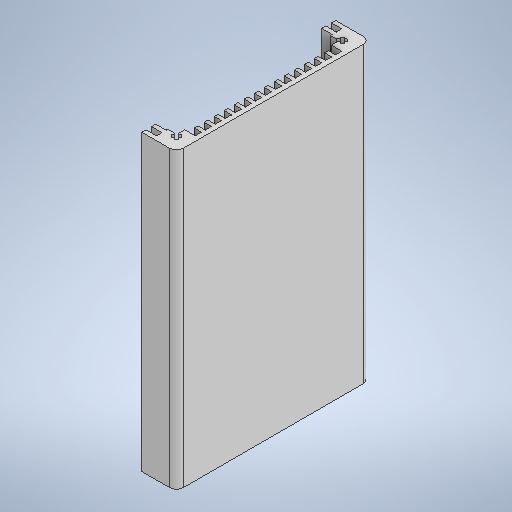
# Autodesk Inventor part: Side Section 2
Saved by Autodesk Inventor 2025 (Build 290162000, 162)
## iProperties
Created: 2024-06-11
Part Number: Side Section 2
Material: Generic
Document SubType Name: Modeling
Designer: Caleb Fangmeier
Density: 1 g/cm^3
Appearance: Default
Author: Caleb Fangmeier
Autodesk Inventor part; units mm, degrees
ref_plane "YZ Plane" through (0, 0, 0) normal (1, 0, 0) x (0, 1, 0)
ref_plane "XZ Plane" through (0, 0, 0) normal (0, 1, 0) x (-1, 0, 0)
ref_plane "XY Plane" through (0, 0, 0) normal (0, 0, 1) x (1, 0, 0)
sketch "Sketch1" plane through (0, 0, 0) normal (0, 1, 0) x (-1, 0, 0)
  line L0 (0, 28) -> (0, -28)
  line L1 (0, 28) -> (10, 28)
  line L2 (0, 28) -> (10, 28) construction
  line L3 (10, 28) -> (10, 26.8)
  line L4 (10, 26.8) -> (7, 26.8)
  line L5 (7, 26.8) -> (7, 25.2)
  line L6 (7, 25.2) -> (10, 25.2)
  line L7 (10, 25.2) -> (10, 24)
  line L8 (10, 24) -> (7, 24)
  line L9 (2.9393, 24.3536) -> (3.6464, 25.0607)
  line L10 (2.9393, 24.3536) -> (3.9393, 24.3536) construction
  line L11 (3.6464, 25.0607) -> (4, 24.7071)
  line L12 (4, 24.7071) -> (4.3536, 25.0607)
  line L13 (4.3536, 25.0607) -> (5.0607, 24.3536)
  line L14 (5.0607, 24.3536) -> (4.7071, 24)
  line L15 (2.9393, 24.3536) -> (3.2929, 24)
  line L16 (3.2929, 24) -> (2.9393, 23.6464)
  line L17 (2.9393, 23.6464) -> (3.6464, 22.9393)
  line L18 (3.6464, 22.9393) -> (4, 23.2929)
  line L19 (4.7071, 24) -> (5.2071, 23.5)
  line L20 (4, 23.2929) -> (4.3536, 22.9393)
  line L21 (7, 24) -> (7, 23.5)
  line L22 (7, 23.5) -> (5.2071, 23.5)
  line L23 (1.4, 0) -> (1.4, 0.9)
  line L24 (1.4, 0.9) -> (3.5, 0.9)
  line L25 (3.5, 0.9) -> (3.5, 2)
  line L26 (3.5, 2) -> (1.4, 2)
  line L27 (1.4, 2) -> (1.4, 2.9)
  line L28 (1.4, 2.9) -> (1.4, 3.8)
  line L29 (1.4, 3.8) -> (3.5, 3.8)
  line L30 (3.5, 3.8) -> (3.5, 4.9)
  line L31 (3.5, 4.9) -> (1.4, 4.9)
  line L32 (1.4, 4.9) -> (1.4, 5.8)
  line L33 (1.4, 5.8) -> (1.4, 6.7)
  line L34 (1.4, 6.7) -> (3.5, 6.7)
  line L35 (3.5, 6.7) -> (3.5, 7.8)
  line L36 (3.5, 7.8) -> (1.4, 7.8)
  line L37 (1.4, 7.8) -> (1.4, 8.7)
  line L38 (1.4, 8.7) -> (1.4, 9.6)
  line L39 (1.4, 9.6) -> (3.5, 9.6)
  line L40 (3.5, 9.6) -> (3.5, 10.7)
  line L41 (3.5, 10.7) -> (1.4, 10.7)
  line L42 (1.4, 10.7) -> (1.4, 11.6)
  line L43 (1.4, 11.6) -> (1.4, 12.5)
  line L44 (1.4, 12.5) -> (3.5, 12.5)
  line L45 (3.5, 12.5) -> (3.5, 13.6)
  line L46 (3.5, 13.6) -> (1.4, 13.6)
  line L47 (1.4, 13.6) -> (1.4, 14.5)
  line L48 (1.4, 14.5) -> (1.4, 15.4)
  line L49 (1.4, 15.4) -> (3.5, 15.4)
  line L50 (3.5, 15.4) -> (3.5, 16.5)
  line L51 (3.5, 16.5) -> (1.4, 16.5)
  line L52 (1.4, 16.5) -> (1.4, 17.4)
  line L53 (1.4, 17.4) -> (1.4, 18.3)
  line L54 (1.4, 18.3) -> (3.5, 18.3)
  line L55 (3.5, 18.3) -> (3.5, 19.4)
  line L56 (3.5, 19.4) -> (1.4, 19.4)
  line L57 (1.4, 19.4) -> (1.4, 20.3)
  line L58 (1.4, 20.3) -> (1.4, 21.2)
  line L59 (1.4, 21.2) -> (4.4, 21.2)
  line L60 (4.4, 21.2) -> (4.4, 22.8929)
  line L61 (4.4, 22.8929) -> (4.3536, 22.9393)
  line L62 (13.8128, 0) -> (-10.738, 0)
  line L63 (0, -28) -> (10, -28)
  line L64 (0, -28) -> (10, -28) construction
  line L65 (10, -28) -> (10, -26.8)
  line L66 (10, -26.8) -> (7, -26.8)
  line L67 (7, -26.8) -> (7, -25.2)
  line L68 (7, -25.2) -> (10, -25.2)
  line L69 (10, -25.2) -> (10, -24)
  line L70 (10, -24) -> (7, -24)
  line L71 (2.9393, -24.3536) -> (3.6464, -25.0607)
  line L72 (2.9393, -24.3536) -> (3.9393, -24.3536) construction
  line L73 (3.6464, -25.0607) -> (4, -24.7071)
  line L74 (4, -24.7071) -> (4.3536, -25.0607)
  line L75 (4.3536, -25.0607) -> (5.0607, -24.3536)
  line L76 (5.0607, -24.3536) -> (4.7071, -24)
  line L77 (2.9393, -24.3536) -> (3.2929, -24)
  line L78 (3.2929, -24) -> (2.9393, -23.6464)
  line L79 (2.9393, -23.6464) -> (3.6464, -22.9393)
  line L80 (3.6464, -22.9393) -> (4, -23.2929)
  line L81 (4.7071, -24) -> (5.2071, -23.5)
  line L82 (4, -23.2929) -> (4.3536, -22.9393)
  line L83 (7, -24) -> (7, -23.5)
  line L84 (7, -23.5) -> (5.2071, -23.5)
  line L85 (1.4, 0) -> (1.4, -0.9)
  line L86 (1.4, -0.9) -> (3.5, -0.9)
  line L87 (3.5, -0.9) -> (3.5, -2)
  line L88 (3.5, -2) -> (1.4, -2)
  line L89 (1.4, -2) -> (1.4, -2.9)
  line L90 (1.4, -2.9) -> (1.4, -3.8)
  line L91 (1.4, -3.8) -> (3.5, -3.8)
  line L92 (3.5, -3.8) -> (3.5, -4.9)
  line L93 (3.5, -4.9) -> (1.4, -4.9)
  line L94 (1.4, -4.9) -> (1.4, -5.8)
  line L95 (1.4, -5.8) -> (1.4, -6.7)
  line L96 (1.4, -6.7) -> (3.5, -6.7)
  line L97 (3.5, -6.7) -> (3.5, -7.8)
  line L98 (3.5, -7.8) -> (1.4, -7.8)
  line L99 (1.4, -7.8) -> (1.4, -8.7)
  line L100 (1.4, -8.7) -> (1.4, -9.6)
  line L101 (1.4, -9.6) -> (3.5, -9.6)
  line L102 (3.5, -9.6) -> (3.5, -10.7)
  line L103 (3.5, -10.7) -> (1.4, -10.7)
  line L104 (1.4, -10.7) -> (1.4, -11.6)
  line L105 (1.4, -11.6) -> (1.4, -12.5)
  line L106 (1.4, -12.5) -> (3.5, -12.5)
  line L107 (3.5, -12.5) -> (3.5, -13.6)
  line L108 (3.5, -13.6) -> (1.4, -13.6)
  line L109 (1.4, -13.6) -> (1.4, -14.5)
  line L110 (1.4, -14.5) -> (1.4, -15.4)
  line L111 (1.4, -15.4) -> (3.5, -15.4)
  line L112 (3.5, -15.4) -> (3.5, -16.5)
  line L113 (3.5, -16.5) -> (1.4, -16.5)
  line L114 (1.4, -16.5) -> (1.4, -17.4)
  line L115 (1.4, -17.4) -> (1.4, -18.3)
  line L116 (1.4, -18.3) -> (3.5, -18.3)
  line L117 (3.5, -18.3) -> (3.5, -19.4)
  line L118 (3.5, -19.4) -> (1.4, -19.4)
  line L119 (1.4, -19.4) -> (1.4, -20.3)
  line L120 (1.4, -20.3) -> (1.4, -21.2)
  line L121 (1.4, -21.2) -> (4.4, -21.2)
  line L122 (4.4, -21.2) -> (4.4, -22.8929)
  line L123 (4.4, -22.8929) -> (4.3536, -22.9393)
  point P0 (0, 0)
  point P1 (4, 24)
  point P2 (0, 0)
  point P3 (4, -24)
  dimension "d0" = 56
  dimension "d1" = 10
  dimension "d3" = 28
  dimension "d4" = 1.2
  dimension "d5" = 3
  dimension "d6" = 1.6
  dimension "d7" = 1.2
  dimension "d9" = 24
  dimension "d10" = 4
  dimension "d11" = 1
  dimension "d12" = 45
  dimension "d13" = 1
  dimension "d14" = 1
  dimension "d15" = 0.5
  dimension "d16" = 0.5
  dimension "d17" = 0.5
  dimension "d18" = 0.5
  dimension "d20" = 0.5
  dimension "d21" = 0.5
  dimension "d25" = 0.9
  dimension "d26" = 1.4
  dimension "d27" = 2.1
  dimension "d28" = 1.1
  dimension "d29" = 0.9
  dimension "d32" = 2.9
  dimension "d37" = 0.9
  dimension "d38" = 3
  constraints: 248 end point, 67 symmetric about line, 15 perpendicular, 10 point on line, 7 vertical, 6 horizontal, 3 vertical alignment, 2 equal length, 2 horizontal alignment, 2 midpoint, 1 parallel, 66 other
  measures "d0" distance of L0.start L0.end
  measures "d1" distance of L0.start L1.end
  measures "d3" distance of L0.start point (0, 0)
  measures "d4" distance of L2.end L3.end
  measures "d5" distance of L3.end L4.end
  measures "d6" distance of L4.end L5.end
  measures "d7" distance of L6.end L7.end
  measures "d9" vertical distance of point (4, 24) point (0, 0)
  measures "d10" horizontal distance of point (0, 0) point (4, 24)
  measures "d11" distance of L9.start L9.end
  measures "d12" angle of L10 L9
  measures "d13" distance of L12.end L13.end
  measures "d14" distance of L16.end L17.end
  measures "d15" distance of L9.start L15.end
  measures "d16" distance of L9.end L11.end
  measures "d17" distance of L13.end L14.end
  measures "d18" distance of L17.end L18.end
  measures "d20" distance of L18.end L20.end
  measures "d21" distance of L8.end L21.end
  measures "d25" distance of L23.start L23.end
  measures "d26" distance between parallel lines of L0 L23
  measures "d27" distance of L23.end L24.end
  measures "d28" distance of L24.end L25.end
  measures "d29" distance of L26.end L27.end
  measures "d32" distance of L23.start L28.start
  measures "d37" distance of L57.end L58.end
  measures "d38" distance of L58.end L59.end
extrude "Extrusion1" add sketch "Sketch1" along normal blind 85
fillet "Fillet1" radius 2 2 edges at (0, 42.5, 28) (0, 42.5, -28)
equation "\"d3\" = 0.5 * d0"
equation "\"d13\" = d11"
equation "\"d14\" = d11"
equation "\"d16\" = d15"
equation "\"d17\" = d15"
equation "\"d18\" = d15"
equation "\"d20\" = d15"
body "Solid1"
